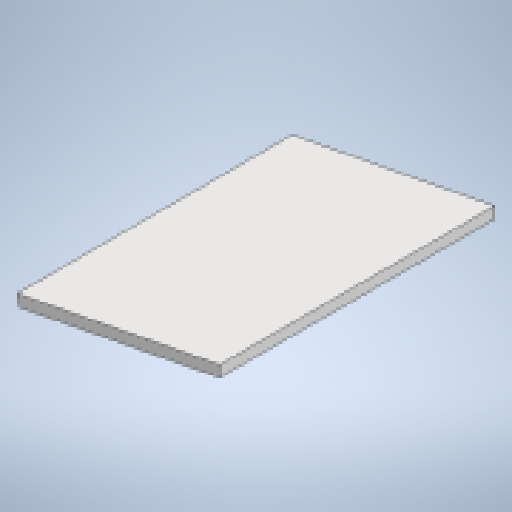
# Autodesk Inventor part: nozzyk
Saved by Autodesk Inventor 2023.5 (Build 275446000, 446)
## iProperties
Created: 2025-03-26
Part Number: nozzyk
Material: Ogólny
Document SubType Name: Modeling
Designer: kamil
Density: 1 g/cm^3
Appearance: Domyślna
Author: kamil
Autodesk Inventor part; units mm, degrees
ref_plane "YZ Plane" through (0, 0, 0) normal (1, 0, 0) x (0, 1, 0)
ref_plane "XZ Plane" through (0, 0, 0) normal (0, 1, 0) x (-1, 0, 0)
ref_plane "XY Plane" through (0, 0, 0) normal (0, 0, 1) x (1, 0, 0)
sketch "Szkic1" plane through (0, 0, 0) normal (0, 0, 1) x (1, 0, 0)
  line L0 (0, 50) -> (-36.8111, 42.8048)
  line L1 (-36.8111, 42.8048) -> (-36.4275, 40.8419)
  line L2 (-36.4275, 40.8419) -> (0, 47.9622)
  line L3 (0, 47.9622) -> (0, 50)
  line L4 (0, 0) -> (0, 50) projected
  point P0 (-25.67, 42.9446)
  dimension "d0" = 2
  constraints: 8 end point, 1 collinear, 1 parallel, 1 perpendicular, 1 point on line, 2 other
  measures "d0" distance between parallel lines of L0 L2
extrude "Wyciągnięcie proste1" add sketch "Szkic1" against normal blind 50
sketch "Szkic2" plane through (0, 50, 0) normal (-0.1918, 0.9814, 0) x (0.9814, 0.1918, 0)
  line L0 (-18.8923, 11.5698) -> (-18.8923, 7.1698) projected
  line L1 (-21.2632, 7.1698) -> (-21.2632, 11.5698) projected
  line L2 (-18.8923, 7.1698) -> (-21.2632, 7.1698) projected
  line L3 (-21.2632, 11.5698) -> (-18.8923, 11.5698) projected
  line L4 (-18.8923, 38.3698) -> (-21.2632, 38.3698) projected
  line L5 (-21.2632, 38.3698) -> (-21.2632, 42.7698) projected
  line L6 (-21.2632, 42.7698) -> (-18.8923, 42.7698) projected
  line L7 (-18.8923, 42.7698) -> (-18.8923, 38.3698) projected
  line L8 (-16.8923, 5.1698) -> (-16.8923, 13.5698)
  line L9 (-16.8923, 13.5698) -> (-23.2632, 13.5698)
  line L10 (-23.2632, 13.5698) -> (-23.2632, 5.1698)
  line L11 (-23.2632, 5.1698) -> (-16.8923, 5.1698)
  line L12 (-16.8923, 36.3698) -> (-23.2632, 36.3698)
  line L13 (-23.2632, 36.3698) -> (-23.2632, 44.7698)
  line L14 (-23.2632, 44.7698) -> (-16.8923, 44.7698)
  line L15 (-16.8923, 44.7698) -> (-16.8923, 36.3698)
  circle A0 centre (-10.1487, 6) radius 1.4 projected
  circle A1 centre (-10.1518, 45) radius 1.4 projected
  point P0 (-9.5917, 0)
  dimension "d3" = 2
  dimension "d4" = 2
  constraints: 16 end point, 6 other
  measures "d3" distance between parallel lines of L0 L8
  measures "d4" distance between parallel lines of L7 L15
extrude "Wyciągnięcie proste2" cut sketch "Szkic2" against normal through all contours L0 L2 L1 L3 | L4 L5 L6 L7 | L11 L10 L9 L8 | L12 L13 L14 L15 | A0 | A1
